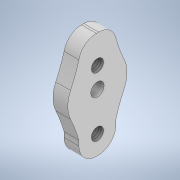
# Autodesk Inventor part: soiya
Saved by Autodesk Inventor 2022 (Build 260153000, 153)
## iProperties
Created: 2022-12-16
Part Number: soiya
Material: 一般
Document SubType Name: Modeling
Designer: tdn82
Density: 1 g/cm^3
Appearance: 既定
Author: tdn82
Autodesk Inventor part; units mm, degrees
ref_plane "YZ Plane" through (0, 0, 0) normal (1, 0, 0) x (0, 1, 0)
ref_plane "XZ Plane" through (0, 0, 0) normal (0, 1, 0) x (-1, 0, 0)
ref_plane "XY Plane" through (0, 0, 0) normal (0, 0, 1) x (1, 0, 0)
sketch "スケッチ1" plane through (0, 0, 0) normal (1, 0, 0) x (0, 1, 0)
  circle A0 centre (0, 0) radius 10
  dimension "d0" = 20
  constraints: 1 centre point, 1 coincident
  measures "d0" diameter of A0
extrude "押し出し1" add sketch "スケッチ1" along normal blind 5
sketch "スケッチ2" plane through (0, 0, 0) normal (-1, 0, 0) x (0, 0, 1)
  circle A0 centre (0, 0) radius 2.25
  dimension "d3" = 4.5
  constraints: 1 centre point, 1 coincident
  measures "d3" diameter of A0
extrude "押し出し2" cut sketch "スケッチ2" against normal through all
sketch "スケッチ3" plane through (0, 0, 0) normal (-1, 0, 0) x (0, 0, 1)
  line L0 (0, -10) -> (0, 10) construction
  line L1 (6.5, -10) -> (6.5, 10)
  line L2 (-6.5, 10) -> (-6.5, -10)
  arc A0 (-6.5, -10) -> (6.5, -10) centre (0, -10) ccw
  arc A1 (6.5, 10) -> (-6.5, 10) centre (0, 10) ccw
  circle A2 centre (0, 0) radius 2.25 projected
  circle A3 centre (0, 0) radius 10 projected
  point P0 (-6.5, 7.5993)
  point P1 (6.5, 7.5993)
  point P2 (6.5, -7.5993)
  point P3 (-6.5, -7.5993)
  dimension "d7" = 13
  constraints: 8 end point, 4 point on circle, 4 tangent, 2 centre point, 2 coincident, 1 midpoint, 1 parallel, 1 vertical
  measures "d7" distance between parallel lines of L1 L2
extrude "押し出し3" add sketch "スケッチ3" against normal up to surface (5 mm away) contours A0 L2 A3 L1 | A3 L2 A1 L1
fillet "フィレット1" radius 50 4 edges at (2.5, -7.5993, 6.5) (2.5, 7.5993, 6.5) (2.5, 7.5993, -6.5) (2.5, -7.5993, -6.5)
sketch "スケッチ4" plane through (0, 0, 0) normal (-1, 0, 0) x (0, 0, 1)
  arc A0 (-6.2543, -11.7702) -> (6.2543, -11.7702) centre (0, -10) ccw projected
  circle A1 centre (0, 0) radius 2.25 projected
  point P0 (0, 7)
  point P1 (0, -13)
  dimension "d22" = 20
  dimension "d23" = 7
  constraints: 1 coincident
  measures "d22" distance of point (0, -13) point (0, 7)
  measures "d23" distance of A1.centre point (0, 7)
hole "穴1" at (0, 7, 0) at (0, -13, 0) direction (1, 0, 0) diameter 4.134 end through all thread size "M5x0.8" class "6H" standard "ISO Metric profile"
sketch "スケッチ6" plane through (0, 0, 0) normal (-1, 0, 0) x (0, 0, 1)
  line L0 (6.2543, -11.7702) -> (6.2543, -19.439)
  line L1 (6.2543, -19.439) -> (-6.2543, -19.439)
  line L2 (-6.2543, -19.439) -> (-6.2543, -11.7702)
  circle A0 centre (0, -10.0493) radius 6.4535
  point P0 (0, 0)
  constraints: 6 end point, 1 centre point, 1 parallel
extrude "押し出し4" add sketch "スケッチ6" against normal blind 5 fills toward (6.2043, -15.6046) open curves L0 L1 L2
fillet "フィレット2" radius 6 1 edges at (2.5, -19.439, -6.2543)
fillet "フィレット3" radius 6 1 edges at (2.5, -19.439, 6.2543)
sketch "スケッチ7" plane through (0, 0, 0) normal (-1, 0, 0) x (0, 0, 1)
  arc A0 (6.2543, 11.7702) -> (-6.2543, 11.7702) centre (0, 10) ccw projected
  line L0 (-6.2543, 11.7702) -> (6.2543, 11.7702)
  line L1 (6.2543, 11.7702) -> (6.2543, 16.5707)
  line L2 (6.2543, 16.5707) -> (-6.2543, 16.5707)
  line L3 (-6.2543, 16.5707) -> (-6.2543, 11.7702)
  point P0 (0, 0)
  constraints: 8 end point, 2 parallel, 1 horizontal, 1 perpendicular
extrude "押し出し5" add sketch "スケッチ7" against normal blind 5 contours A0 L3 L2 L1
fillet "フィレット4" radius 6 1 edges at (2.5, 16.5707, 6.2543)
fillet "フィレット5" radius 6 1 edges at (2.5, 16.5707, -6.2543)
